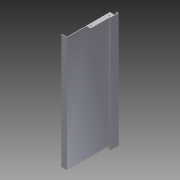
# Autodesk Inventor part: bok szuflady metalbox 150x400mm prawy
Saved by Autodesk Inventor 2013 (Build 170138000, 138)
## iProperties
Created: 2014-05-20
Part Number: bok szuflady metalbox 150x400mm prawy
Material: Ogólny
Document SubType Name: Modeling
Designer: Piotr
Density: 1 g/cm^3
Author: Piotr
Autodesk Inventor part; units mm, degrees
ref_plane "YZ Plane" through (0, 0, 0) normal (1, 0, 0) x (0, 1, 0)
ref_plane "XZ Plane" through (0, 0, 0) normal (0, 1, 0) x (-1, 0, 0)
ref_plane "XY Plane" through (0, 0, 0) normal (0, 0, 1) x (1, 0, 0)
sketch "Szkic1" plane through (0, 0, 0) normal (0, 0, 1) x (1, 0, 0)
  line L0 (0, 0) -> (17, 0)
  line L1 (17, 0) -> (17, -2)
  line L2 (17, -2) -> (-2, -2)
  line L3 (-2, -2) -> (-2, 148)
  line L4 (-2, 148) -> (-16, 148)
  line L5 (-16, 148) -> (-16, 150)
  line L6 (-16, 150) -> (0, 150)
  line L7 (0, 150) -> (0, 0)
  line L8 (0, 150) -> (17, 150)
  line L9 (17, 150) -> (17, 0)
  line L10 (-16, 150) -> (-16, 160)
  line L11 (-16, 160) -> (-10, 160)
  line L12 (-10, 160) -> (-10, 162)
  line L13 (-10, 162) -> (-18, 162)
  line L14 (-18, 162) -> (-18, 135)
  line L15 (-18, 135) -> (-10, 135)
  line L16 (-10, 135) -> (-10, 137)
  line L17 (-10, 137) -> (-16, 137)
  line L18 (-16, 137) -> (-16, 148)
  dimension "d0" = 17
  dimension "d1" = 2
  dimension "d2" = 2
  dimension "d3" = 148
  dimension "d4" = 2
  dimension "d5" = 14
  dimension "d10" = 2
  dimension "d11" = 6
  dimension "d12" = 2
  dimension "d13" = 2
  dimension "d14" = 27
  dimension "d15" = 11
  constraints: 38 end point, 13 parallel, 5 perpendicular, 1 collinear, 1 horizontal
  measures "d0" distance of L0.start L0.end
  measures "d1" distance of L0.end L1.end
  measures "d2" distance of L4.end L5.end
  measures "d3" distance between parallel lines of L0 L4
  measures "d4" distance between parallel lines of L7 L3
  measures "d5" distance of L3.end L4.end
  measures "d10" distance of L11.end L12.end
  measures "d11" distance of L16.end L17.end
  measures "d12" distance between parallel lines of L14 L10
  measures "d13" distance of L15.end L16.end
  measures "d14" distance of L13.end L14.end
  measures "d15" distance of L17.end L4.end
extrude "Wyciągnięcie proste1" add sketch "Szkic1" along normal blind 400 contours L0 L1 L2 L3 L4 L5 L6 L7 | L5 L18 L17 L16 L15 L14 L13 L12 L11 L10
extrude "Wyciągnięcie proste2" add sketch "Szkic1" along normal blind 2 contours L7 L8 L9 L0
sketch "Szkic2" plane through (0, 0, 400) normal (0, 0, 1) x (1, 0, 0)
  line L0 (-16, 148) -> (-2, 148) projected
  line L1 (-2, 148) -> (-2, -2) projected
  line L2 (17, 0) -> (0, 0) projected
  line L3 (-16, 148) -> (-2, 148)
  line L4 (-2, 148) -> (-2, 67)
  line L5 (-2, 67) -> (-16, 67)
  line L6 (-16, 67) -> (-16, 148)
  line L7 (-9, 67) -> (-9, 148) construction
  point P0 (-9, 75)
  point P1 (-9, 139)
  dimension "d16" = 75
  dimension "d17" = 64
  dimension "d18" = 8
  constraints: 10 end point, 3 point on line, 2 midpoint, 2 parallel, 1 horizontal, 1 perpendicular
  measures "d16" distance from line of point (-9, 75) L2
  measures "d17" distance of point (-9, 75) point (-9, 139)
  measures "d18" distance from line of L5 point (-9, 75)
extrude "Wyciągnięcie proste3" add sketch "Szkic2" against normal blind 2
hole "Otwór1" at (-9, 75, 400) at (-9, 139, 400) direction (0, 0, -1) diameter 4 end up to surface
mirror "Odbicie lustrzane1" about plane through (0, 0, 0) normal (1, 0, 0) remove original yes
